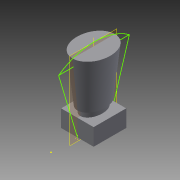
# Autodesk Inventor part: MalePassengerTL
Saved by Autodesk Inventor 2015 (Build 190159000, 159)
## iProperties
Created: 2015-03-13
Part Number: MalePassengerTL
Material: Generic
Document SubType Name: Modeling
Designer: PLTW-Stu-02
Density: 1 g/cm^3
Appearance: Default
Author: PLTW-Stu-02
Autodesk Inventor part; units mm, degrees
ref_plane "YZ Plane" through (0, 0, 0) normal (1, 0, 0) x (0, 1, 0)
ref_plane "XZ Plane" through (0, 0, 0) normal (0, 1, 0) x (-1, 0, 0)
ref_plane "XY Plane" through (0, 0, 0) normal (0, 0, 1) x (1, 0, 0)
sketch "Sketch2" plane through (0, 0, 0) normal (0, 1, 0) x (-1, 0, 0)
  line L0 (25.7555, -11.7629) -> (11.1505, -11.7629)
  line L1 (11.1505, -11.7629) -> (11.1505, -26.3679)
  line L2 (11.1505, -26.3679) -> (25.7555, -26.3679)
  line L3 (25.7555, -26.3679) -> (25.7555, -11.7629)
  point P0 (0, 0)
  dimension "d0" = 14.605
  dimension "d1" = 14.605
  constraints: 8 end point, 2 parallel, 1 horizontal, 1 perpendicular
  measures "d0" distance of L2.end L1.end
  measures "d1" distance of L1.end L0.end
extrude "Extrusion1" add sketch "Sketch2" along normal blind 7.62
sketch "Sketch3" plane through (0, 7.62, 0) normal (0, 1, 0) x (1, 0, 0)
  ellipse E0 centre (-18.453, 19.0654) end of major axis (-18.453, 25.0598) minor radius 3.937
  ellipse E1 centre (-18.453, 19.0654) end of major axis (-18.453, 26.3298) minor radius 5.207
  point P0 (0, 0)
  dimension "d13" = 5.9944
  dimension "d14" = 3.937
  dimension "d15" = 5.207
  dimension "d16" = 7.2644
  constraints: 1 coincident, 4 other
extrude "Extrusion3" add sketch "Sketch3" along normal blind 2.794 contours E0
sketch "Sketch6" plane through (0, 10.414, 0) normal (0, 1, 0) x (1, 0, 0)
  ellipse E0 centre (-18.453, 19.0654) end of major axis (-18.453, 26.3298) minor radius 5.207 projected
  ellipse E1 centre (-18.453, 19.0654) end of major axis (-18.453, 13.071) minor radius 3.937 projected
  ellipse E2 centre (-18.453, 19.0654) end of major axis (-18.453, 26.3298) minor radius 5.207
  point P0 (0, 0)
  constraints: 1 coincident, 4 other
extrude "Extrusion4" add sketch "Sketch6" along normal blind 21.336 draft 6 contours E0 | E1
ref_plane "Work Plane2" through (-18.453, 0, -11.7629) normal (1, 0, 0) x (0, 0, -1)
sketch "Sketch9" plane through (-18.453, 0, -11.7629) normal (1, 0, 0) x (0, 0, -1)
  arc A0 (23.2608, 28.3606) -> (-8.4979, 28.3606) centre (7.3815, 6.1892) ccw
  line L0 (-8.4979, 28.3606) -> (23.2608, 28.3606)
  line L1 (23.2608, 28.3606) -> (14.605, 0)
  line L2 (14.605, 0) -> (0, 0)
  line L3 (14.605, 0) -> (0, 0) projected
  line L4 (0, 0) -> (-8.4979, 28.3606)
  point P0 (-11.7629, 0)
  constraints: 8 end point, 2 point on circle, 1 centre point, 1 collinear, 1 horizontal
body "Solid1"
